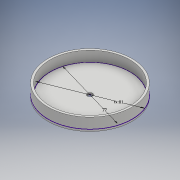
# Autodesk Inventor part: Cap
Saved by Autodesk Inventor 2017 (Build 210142000, 142)
## iProperties
Created: 2016-05-10
Part Number: Cap
Material: Generic
Document SubType Name: Modeling
Designer: Bastli
Density: 1 g/cm^3
Appearance: Default
Author: Bastli
Autodesk Inventor part; units mm, degrees
ref_plane "YZ Plane" through (0, 0, 0) normal (1, 0, 0) x (0, 1, 0)
ref_plane "XZ Plane" through (0, 0, 0) normal (0, 1, 0) x (-1, 0, 0)
ref_plane "XY Plane" through (0, 0, 0) normal (0, 0, 1) x (1, 0, 0)
sketch "Sketch1" plane through (0, 0, 0) normal (0, 0, 1) x (1, 0, 0)
  circle A0 centre (0, 0) radius 38.5
  circle A1 centre (0, 0) radius 40.5
  dimension "Inner_Diameter" = 77
  dimension "d1" = 81
  constraints: 2 centre point, 2 coincident
  measures "Inner_Diameter" diameter of A0
  measures "d1" diameter of A1
extrude "Extrusion1" add sketch "Sketch1" against normal blind 2 contours A0 | A1
extrude "Extrusion2" add sketch "Sketch1" along normal blind 10
sketch "Sketch2" plane through (0, 0, -2) normal (0, 0, -1) x (-1, 0, 0)
  circle A0 centre (0, 0) radius 2.5
  dimension "Axis_Hole" = 5
  constraints: 1 centre point, 1 coincident
  measures "Axis_Hole" diameter of A0
extrude "Extrusion3" cut sketch "Sketch2" against normal up to surface (2 mm away) from surface at 0
equation "\"d1\" = Inner_Diameter + 2 * Thickness"
equation "\"Thickness\" = 2"
body "Solid1"
